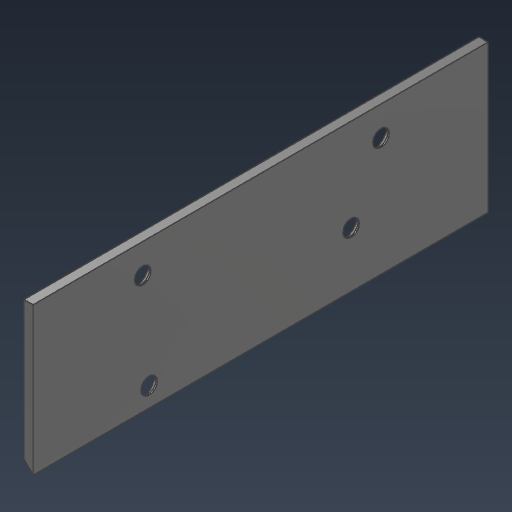
# Autodesk Inventor part: back
Saved by Autodesk Inventor 2023 (Build 270158000, 158)
## iProperties
Created: 2025-03-30
Part Number: back
Material: Aluminum 6061
Document SubType Name: Modeling
Designer: szymo
Density: 2.7 g/cm^3
Appearance: Anodized - Light Gray
Mass: 16.1772 g
Surface Area: 67.3733 cm^2
Volume: 5.99157 cm^3
Author: szymo
Autodesk Inventor part; units mm, degrees
ref_plane "YZ Plane" through (0, 0, 0) normal (1, 0, 0) x (0, 1, 0)
ref_plane "XZ Plane" through (0, 0, 0) normal (0, 1, 0) x (-1, 0, 0)
ref_plane "XY Plane" through (0, 0, 0) normal (0, 0, 1) x (1, 0, 0)
sketch "Sketch1" plane through (0, 0, 0) normal (1, 0, 0) x (0, 1, 0)
  line L0 (-1.5444, -22.1086) -> (30.5556, -22.1086)
  line L1 (30.5556, -22.1086) -> (30.5556, 76.8914)
  line L2 (30.5556, 76.8914) -> (-1.5444, 76.8914)
  line L3 (-1.5444, 76.8914) -> (-1.5444, -22.1086)
  line L4 (28.5556, 60.8914) -> (28.5556, -2.6086) projected
  line L5 (-0.0444, -4.4086) -> (-1.5444, -4.4086) projected
  line L6 (-0.0444, 59.1914) -> (-1.5444, 59.1914) projected
  dimension "d0" = 32.1
  dimension "d1" = 99
  dimension "d21" = 2
  dimension "d22" = 0
  dimension "d23" = 17.7
  dimension "d24" = 17.7
  constraints: 8 end point, 2 parallel, 1 horizontal, 1 perpendicular
  measures "d0" distance of L2.end L1.end
  measures "d1" distance of L1.end L0.end
  measures "d21" distance between parallel lines of L1 L4
  measures "d22" distance from line of L5.end L3
  measures "d23" distance between parallel lines of L0 L5
  measures "d24" distance between parallel lines of L2 L6
extrude "Extrusion1" add sketch "Sketch1" against normal blind 2
sketch "Sketch3" plane through (0, -1.5444, 76.8914) normal (0, 0, 1) x (1, 0, 0)
  line L0 (0, 32.1) -> (0, 0) projected
  line L1 (0, 32.1) -> (-2, 32.1) projected
  line L2 (-2, 0) -> (-2, 32.1) projected
  line L3 (0, 0) -> (-2, 0) projected
  line L4 (0, 0) -> (-2, 0) projected
  line L5 (0, 0) -> (-2, 2)
  line L6 (-2, 32.1) -> (-2, 0) projected
  point P0 (0, 1.5444)
  dimension "d17" = 45
  constraints: 2 end point, 1 point on line
  measures "d17" angle of L0 L5
extrude "Extrusion2" cut sketch "Sketch3" against normal up to surface (99 mm away) contours L3 L2 L5
sketch "Sketch4" plane through (-2, 0, 0) normal (-1, 0, 0) x (0, 0, 1)
  circle A0 centre (7.6914, 10.4556) radius 2.5 projected
  line L0 (11.1914, 27.6556) -> (11.1914, -0.0444) projected
  line L1 (11.1914, 27.6556) -> (-2.4086, 27.6556) projected
  line L2 (11.1914, -0.0444) -> (-2.4086, -0.0444) projected
  circle A1 centre (51.6414, 2.7056) radius 2.5 projected
  circle A2 centre (53.0414, 24.1556) radius 2.5 projected
  line L3 (48.8914, 27.6556) -> (48.8914, -0.0444) projected
  line L4 (48.8914, -0.0444) -> (57.1914, -0.0444) projected
  line L5 (48.8914, 27.6556) -> (57.1914, 27.6556) projected
  line L6 (-2.4086, -0.0444) -> (-2.4086, 27.6556) projected
  line L7 (57.1914, 27.6556) -> (57.1914, -0.0444) projected
  circle A3 centre (1.1914, 24.1556) radius 2.5 projected
  point P0 (0, 0)
  point P1 (1.1914, 24.1556)
  point P2 (7.6914, 10.4556)
  point P3 (53.0414, 24.1556)
  point P4 (51.6414, 2.7056)
  constraints: 3 coincident
hole "Hole2" at (-2, 24.1556, 1.1914) at (-2, 10.4556, 7.6914) at (-2, 24.1556, 53.0414) at (-2, 2.7056, 51.6414) direction (1, 0, 0) diameter 3.6 end through all countersink diameter 7 countersink angle 90 clearance for "Countersunk Flat Head Screw ISO 2009/7046" size "M3" standard "ISO"
equation "\"d23\" = d24"
body "Solid1"
